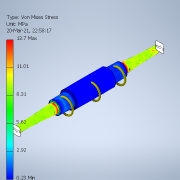
# Autodesk Inventor part: A Shaft
Saved by Autodesk Inventor 2021 (Build 250183000, 183)
## iProperties
Created: 2021-03-20
Part Number: A Shaft
Material: Stainless Steel, 440C
Document SubType Name: Modeling
Designer: TieuBinh
Density: 7.75 g/cm^3
Appearance: Semi-Polished
Author: TieuBinh
Autodesk Inventor part; units mm, degrees
ref_plane "YZ Plane" through (0, 0, 0) normal (1, 0, 0) x (0, 1, 0)
ref_plane "XZ Plane" through (0, 0, 0) normal (0, 1, 0) x (-1, 0, 0)
ref_plane "XY Plane" through (0, 0, 0) normal (0, 0, 1) x (1, 0, 0)
sketch "Sketch1" plane through (0, 0, 0) normal (0, 0, 1) x (1, 0, 0)
  circle A0 centre (0, 0) radius 250
  dimension "d0" = 500
  constraints: 1 centre point, 1 coincident
  measures "d0" diameter of A0
extrude "Extrusion1" add sketch "Sketch1" along normal blind 1000
sketch "Sketch2" plane through (0, 0, 1000) normal (0, 0, 1) x (1, 0, 0)
  circle A0 centre (0, 0) radius 200
  dimension "d3" = 400
  constraints: 1 centre point, 1 coincident
  measures "d3" diameter of A0
extrude "Extrusion2" add sketch "Sketch2" along normal blind 700
sketch "Sketch3" plane through (0, 0, 1700) normal (0, 0, 1) x (1, 0, 0)
  circle A0 centre (0, 0) radius 200 projected
  circle A1 centre (0, 0) radius 150
  dimension "d6" = 300
  constraints: 1 centre point, 1 coincident
  measures "d6" diameter of A1
extrude "Extrusion3" add sketch "Sketch3" along normal blind 2000 contours A1
mirror "Mirror1" about plane through (0, 0, 0) normal (0, 0, -1) of "Extrusion3", "Extrusion2", "Extrusion1"
body "Solid1"
